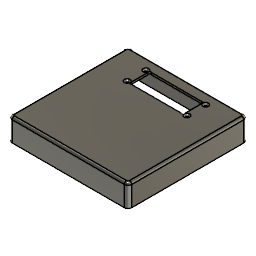
opening for DF Robert 1602 LCD O1002 (Autodesk Fusion 360 archive; units mm, degrees)
design "opening for DF Robert 1602 LCD"
part number: 2026-07-13-18-12-07-008
Autodesk Fusion 360 part; units mm, degrees
sketch "Sketch1" plane through (0, 0, 0) normal (0, 0, 1) x (1, 0, 0)
  line L0 (0, 0) -> (160, 0)
  line L1 (160, 0) -> (160, 160)
  line L2 (160, 160) -> (0, 160)
  line L3 (0, 160) -> (0, 0)
  dimension "d1" = 160
  dimension "d3" = 160
  constraint horizontal L0
  constraint vertical L1
  constraint horizontal L2
  constraint vertical L3
  constraint coincident L0.start L3.end
  measures "d1" distance of L0.start L0.end
  measures "d3" distance of L0.end L1.end
extrude "Extrude1" add sketch "Sketch1" along normal blind 30
fillet "Fillet1" radius 5 4 edges at (0, 160, 15) (0, 0, 15) (160, 0, 15) (160, 160, 15)
fillet "Fillet1" radius 3 4 edges at (160, 80, 30) (80, 160, 30) (80, 0, 30) (0, 80, 30)
shell "Shell1" thickness 2.7 removed faces 1 at (53.3333, 51.6667, 0)
sketch "Sketch3" plane through (0, 0, 30) normal (0, 0, 1) x (-1, 0, 0)
  arc A0 (-5, -157) -> (-3, -155) centre (-5, -155) ccw
  line L0 (-3, -155) -> (-3, -5)
  arc A1 (-3, -5) -> (-5, -3) centre (-5, -5) ccw
  line L1 (-5, -3) -> (-155, -3)
  arc A2 (-155, -3) -> (-157, -5) centre (-155, -5) ccw
  line L2 (-157, -5) -> (-157, -155)
  arc A3 (-157, -155) -> (-155, -157) centre (-155, -155) ccw
  line L3 (-155, -157) -> (-5, -157)
  line L4 (-44, -145) -> (-116, -145)
  line L5 (-116, -145) -> (-116, -118)
  line L6 (-116, -118) -> (-44, -118)
  line L7 (-44, -118) -> (-44, -145)
  arc A4 (-155, 0) -> (-160, -5) centre (-155, -5) ccw
  line L8 (-160, -5) -> (-160, -155)
  arc A5 (-160, -155) -> (-155, -160) centre (-155, -155) ccw
  line L9 (-155, -160) -> (-5, -160)
  arc A6 (-5, -160) -> (0, -155) centre (-5, -155) ccw
  line L10 (0, -155) -> (0, -5)
  arc A7 (0, -5) -> (-5, 0) centre (-5, -5) ccw
  line L11 (-5, 0) -> (-155, 0)
  line L12 (-80, -145) -> (-80, -160) construction
  dimension "d11" = 72
  dimension "d12" = 27
  dimension "d13" = 15
  constraint horizontal L4
  constraint vertical L5
  constraint horizontal L6
  constraint vertical L7
  constraint midpoint L4 L12.start
  constraint midpoint L9 L12.end
  constraint vertical L12
  measures "d11" distance of L4.start L4.end
  measures "d12" distance of L4.start L6.end
  measures "d13" distance of L4 L9
extrude "Extrude2" cut sketch "Sketch3" along normal through all and the other way through all contours L4 L5 L6 L7
sketch "Sketch4" plane through (0, 0, 30) normal (0, 0, 1) x (-1, 0, 0)
  line L0 (-44, -145) -> (-44, -118)
  line L1 (-44, -118) -> (-116, -118)
  line L2 (-116, -118) -> (-116, -145)
  line L3 (-116, -145) -> (-44, -145)
  arc A0 (-155, 0) -> (-160, -5) centre (-155, -5) ccw
  line L4 (-160, -5) -> (-160, -155)
  arc A1 (-160, -155) -> (-155, -160) centre (-155, -155) ccw
  line L5 (-155, -160) -> (-5, -160)
  arc A2 (-5, -160) -> (0, -155) centre (-5, -155) ccw
  line L6 (0, -155) -> (0, -5)
  arc A3 (0, -5) -> (-5, 0) centre (-5, -5) ccw
  line L7 (-5, 0) -> (-155, 0)
  line L8 (-40, -144) -> (-120, -144)
  line L9 (-120, -144) -> (-120, -119)
  line L10 (-120, -119) -> (-40, -119)
  line L11 (-40, -119) -> (-40, -144)
  line L12 (-44, -131.5) -> (-40, -131.5)
  line L13 (-80, -144) -> (-80, -145)
  line L14 (-80, -118) -> (-80, -119)
  line L15 (-116, -131.5) -> (-120, -131.5)
  dimension "d31" = 80
  dimension "d32" = 25
  constraint horizontal L8
  constraint vertical L9
  constraint horizontal L10
  constraint vertical L11
  constraint midpoint L0 L12.start
  constraint midpoint L11 L12.end
  constraint midpoint L8 L13.start
  constraint midpoint L3 L13.end
  constraint coincident L1 L14.start
  constraint coincident L10 L14.end
  constraint parallel L13 L14
  constraint midpoint L10 L14.end
  constraint midpoint L1 L14.start
  constraint midpoint L2 L15.start
  constraint midpoint L9 L15.end
  constraint vertical L13
  constraint horizontal L12
  measures "d31" distance of L8.start L8.end
  measures "d32" distance of L8.start L10.end
sketch "Sketch5" plane through (0, 0, 30) normal (0, 0, 1) x (-1, 0, 0)
  line L0 (-44, -118) -> (-44, -145)
  line L1 (-44, -145) -> (-116, -145)
  line L2 (-116, -145) -> (-116, -118)
  line L3 (-116, -118) -> (-44, -118)
  arc A0 (-5, -157) -> (-3, -155) centre (-5, -155) ccw
  line L4 (-3, -155) -> (-3, -5)
  arc A1 (-3, -5) -> (-5, -3) centre (-5, -5) ccw
  line L5 (-5, -3) -> (-155, -3)
  arc A2 (-155, -3) -> (-157, -5) centre (-155, -5) ccw
  line L6 (-157, -5) -> (-157, -155)
  arc A3 (-157, -155) -> (-155, -157) centre (-155, -155) ccw
  line L7 (-155, -157) -> (-5, -157)
  circle A4 centre (-45.1225, -143.8775) radius 1.5875
  line L8 (-44, -145) -> (-45.1225, -143.8775)
  circle A5 centre (-114.8775, -143.8775) radius 1.5875
  line L9 (-116, -145) -> (-114.8775, -143.8775) construction
  dimension "d23" = 3.175
  dimension "d24" = 45
  dimension "d25" = 3.175
  constraint coincident L0.end A4
  constraint coincident L0.end L1.start
  constraint coincident A4.centre L8.end
  constraint coincident L1.end A5
  constraint coincident L1.end L2.start
  constraint coincident A5.centre L9.end
  measures "d23" diameter of A4
  measures "d24" angle of L1 L8
  measures "d25" diameter of A5
extrude "Extrude3" cut sketch "Sketch5" along normal through all and the other way through all contours L0 A4 | L0 L1 A4 | L1 A4 | L1 L2 A5 | L2 A5 | L1 A5
ref_plane "WorkPlane1" through (80, 131.5, 28.65) normal (0, -1, 0) x (-1, 0, 0)
mirror "Mirror1" about plane through (80, 131.5, 28.65) normal (0, -1, 0) of "Extrude3"
fillet "Fillet2" [suppressed]
hole "Hole1" at (120, 144, 30) at (120, 119, 30) at (40, 119, 30) at (40, 144, 30) direction (0, 0, -1) diameter 3.4 depth 15 tip angle 118 countersink diameter 7.5 countersink angle 90
equation "d1 = Lid_X"
equation "d3 = Lid_Y"
equation "d4 = Lid_Z"
equation "d8 = Lid_Thikness"
equation "d11 = Opening_X"
equation "d12 = Opening_Y"
equation "d23 = d25"
equation "d25 = dog_bone_DIA"
equation "d30 = Corner_rad"
equation "d31 = Holes_X"
equation "d32 = Holes_Y"
equation "Lid_X = 160 mm"
equation "Lid_Y = 160 mm"
equation "Lid_Z = 30 mm"
equation "Opening_X = 72 mm"
equation "Opening_Y = 27 mm"
equation "Lid_Thikness = 2.7 mm"
equation "Corner_rad = 0.793 mm"
equation "Holes_X = 80 mm"
equation "Holes_Y = 25 mm"
equation "dog_bone_DIA = 0'- 1/8\""
